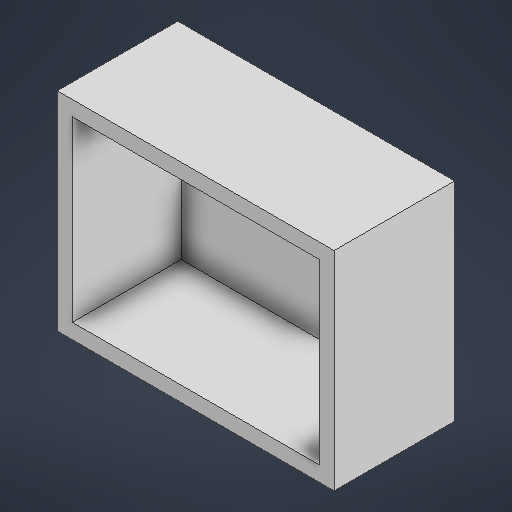
# Autodesk Inventor part: microphone_casing
Saved by Autodesk Inventor 2026 (Build 300175050, 175E)
## iProperties
Created: 2025-06-09
Part Number: microphone_casing
Material: Generic
Document SubType Name: Modeling
Designer: satom
Density: 1 g/cm^3
Appearance: Default
Author: satom
Autodesk Inventor part; units mm, degrees
ref_plane "YZ Plane" through (0, 0, 0) normal (1, 0, 0) x (0, 1, 0)
ref_plane "XZ Plane" through (0, 0, 0) normal (0, 1, 0) x (-1, 0, 0)
ref_plane "XY Plane" through (0, 0, 0) normal (0, 0, 1) x (1, 0, 0)
sketch "Sketch1" plane through (0, 0, 0) normal (0, 0, 1) x (1, 0, 0)
  line L0 (0, 0) -> (23.33, 0)
  line L1 (23.33, 0) -> (23.33, 17.54)
  line L2 (23.33, 17.54) -> (0, 17.54)
  line L3 (0, 17.54) -> (0, 0)
  dimension "d0" = 23.33
  dimension "d1" = 17.54
  constraints: 8 end point, 2 parallel, 1 horizontal, 1 perpendicular
  measures "d0" distance of L1.end L2.end
  measures "d1" distance of L0.end L1.end
extrude "Extrusion1" add sketch "Sketch1" along normal blind 10.16
sketch "Sketch2" plane through (0, 0, 10.16) normal (0, 0, 1) x (1, 0, 0)
  line L0 (1.27, 16.27) -> (22.06, 16.27)
  line L1 (22.06, 16.27) -> (22.06, 1.27)
  line L2 (22.06, 1.27) -> (1.27, 1.27)
  line L3 (1.27, 1.27) -> (1.27, 16.27)
  line L4 (0, 0) -> (23.33, 0) projected
  line L5 (23.33, 0) -> (23.33, 17.54) projected
  line L6 (23.33, 17.54) -> (0, 17.54) projected
  line L7 (0, 17.54) -> (0, 0) projected
  dimension "d4" = 1.27
  dimension "d5" = 1.27
  dimension "d6" = 1.27
  dimension "d7" = 1.27
  constraints: 8 end point, 2 parallel, 1 horizontal, 1 perpendicular
  measures "d4" distance between parallel lines of L4 L2
  measures "d5" distance between parallel lines of L5 L1
  measures "d6" distance between parallel lines of L6 L0
  measures "d7" distance between parallel lines of L7 L3
extrude "Extrusion2" cut sketch "Sketch2" against normal blind 9.16 contours L0 L1 L2 L3
sketch "Sketch3" plane through (0, 0, 1) normal (0, 0, 1) x (1, 0, 0)
  line L0 (23.33, 17.54) -> (0, 17.54) construction
  line L1 (11.665, 17.54) -> (11.665, 0) construction
  line L2 (0, 0) -> (23.33, 0) construction
  line L3 (23.33, 0) -> (23.33, 17.54) construction
  line L4 (23.33, 8.77) -> (0, 8.77) construction
  line L5 (0, 17.54) -> (0, 0) construction
  circle A0 centre (5.115, 12.52) radius 1.7
  circle A1 centre (12.96, 10.66) radius 0.5
  circle A2 centre (18.215, 12.52) radius 1.7
  line L6 (1.27, 16.27) -> (22.06, 16.27) projected
  dimension "d10" = 3.4
  dimension "d11" = 3.4
  dimension "d13" = 6.55
  dimension "d14" = 6.55
  dimension "d15" = 3.75
  dimension "d16" = 3.75
  dimension "d17" = 1
  dimension "d18" = 5.255
  dimension "d19" = 1.86
  constraints: 4 end point, 4 midpoint, 3 centre point, 1 horizontal, 1 vertical
  measures "d10" diameter of A0
  measures "d11" diameter of A2
  measures "d13" distance from line of L1 A0.centre
  measures "d14" distance from line of L1 A2.centre
  measures "d15" distance from line of L6 A0.centre
  measures "d16" distance from line of L6 A2.centre
  measures "d17" diameter of A1
  measures "d18" horizontal distance of A2.centre A1.centre
  measures "d19" vertical distance of A1.centre A2.centre
extrude "Extrusion3" cut sketch "Sketch3" against normal through all
equation "\"d5\" = d4"
equation "\"d6\" = d4"
equation "\"d7\" = d4"
equation "\"d10\" = m3_clearance"
equation "\"d11\" = d12"
equation "\"d14\" = d13"
equation "\"d16\" = d15"
equation "\"m3_heat_set_insert\" = 4"
equation "\"m3_clearance\" = 3.4"
equation "\"m3_heat_set_depth\" = 7"
equation "\"robot_diameter\" = 354"
equation "\"hardboard_thickness\" = 5"
equation "\"d12\" = 3.4"
body "Solid1"
